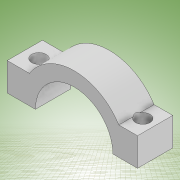
# Autodesk Inventor part: SoporteMotorCierre
Saved by Autodesk Inventor 2022 (Build 260153000, 153)
## iProperties
Created: 2022-03-04
Part Number: SoporteMotorCierre
Material: Genérico
Document SubType Name: Modeling
Designer: Marco
Density: 1 g/cm^3
Appearance: Valor por defecto
Author: Marco
Autodesk Inventor part; units mm, degrees
ref_plane "YZ Plane" through (0, 0, 0) normal (1, 0, 0) x (0, 1, 0)
ref_plane "XZ Plane" through (0, 0, 0) normal (0, 1, 0) x (-1, 0, 0)
ref_plane "XY Plane" through (0, 0, 0) normal (0, 0, 1) x (1, 0, 0)
sketch "Boceto1" plane through (0, 0, 0) normal (0, 0, 1) x (1, 0, 0)
  line L0 (0, 0) -> (8, 0)
  line L1 (30, 0) -> (37, 0)
  arc A0 (30, 0) -> (8, 0) centre (19, 0) ccw
  line L2 (0, 0) -> (0, 8)
  line L3 (0, 8) -> (6.3114, 8)
  line L4 (37, 0) -> (37, 8)
  line L5 (37, 8) -> (31.6886, 8)
  arc A1 (31.6886, 8) -> (6.3114, 8) centre (19, 0) ccw
  line L6 (19, 11) -> (19, 15) construction
  dimension "d0" = 11
  dimension "d1" = 37
  dimension "d2" = 8
  dimension "d3" = 8
  dimension "d5" = 4
  constraints: 14 end point, 6 point on circle, 3 horizontal alignment, 2 centre point, 2 horizontal, 2 perpendicular, 2 vertical, 1 coincident
  measures "d0" radius of A0
  measures "d1" distance of L1.end L0.start
  measures "d2" distance of L0.start L0.end
  measures "d3" distance of L0.start L2.end
  measures "d5" distance of L6.start L6.end
extrude "Extrusión1" add sketch "Boceto1" along normal blind 10
sketch "Boceto3" plane through (0, 0, 0) normal (0, -1, 0) x (1, 0, 0)
  line L0 (0, 0) -> (8, 0) projected
  line L1 (0, 0) -> (0, 10) projected
  line L2 (30, 0) -> (30, 10) projected
  line L3 (30, 0) -> (37, 0) projected
  circle A0 centre (4, 5) radius 2.05
  circle A1 centre (33.5, 5) radius 2.05
  point P0 (0, 5)
  point P1 (30, 5)
  point P2 (4, 0)
  point P3 (33.5, 0)
  dimension "d12" = 4.1
  dimension "d13" = 4.1
  constraints: 4 midpoint, 2 centre point, 2 horizontal alignment, 2 vertical alignment
  measures "d12" diameter of A0
  measures "d13" diameter of A1
extrude "Extrusión3" cut sketch "Boceto3" against normal through all
